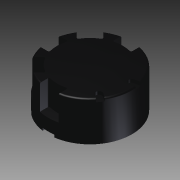
# Autodesk Inventor part: HS13Z-body
Saved by Autodesk Inventor 2011 SP1 (Build 150282100, 282)
## iProperties
Created: 2016-09-01
Part Number: HS13Z-body
Catalog Web Link: www.cadenas.de
Description: HS Series - 6 AMP Single Pole Standard Size Rotaries -body-
Vendor: NKKSWITCHES
Document SubType Name: Modeling
Designer: psAdmin
Manufacturer: NKKSWITCHES
Mass: 13.0423 g
Surface Area: 39.466 cm^2
Volume: 13.0423 cm^3
Density: 1 g/cm^3
Category: PARTsolutions
Company: NKKSWITCHES
Title: HS13Z-body
Author: Cadenas PARTsolutions
PSOL_IDENT_0: {$CADENAS_DATA\23d-libs\nkkswitches\rotary\hs_12_amp\parts\hs_6amp_body.prj},214 {VTYP=3D},{NB=HS13Z
PSOL_IDENT_1: -body},{LINA=HS13Z-body},{NN=HS Series - 6 AMP Single Pole Standard Size Rotaries -body},{DATE=22.09
PSOL_IDENT_2: .2015 06:04:15},{GEOMDATE=26.03.2009 11:48:00},{VERSION=},{LINEID=30},{LINESUBID=-1},{WBVAR=}  {NB=H
PSOL_IDENT_3: S13Z-body},{LINA=HS13Z-body},{KT=DUMMY},{PN=HS13Z},{SRS=HS},{MDL=HS13Z}
NN: HS Series - 6 AMP Single Pole Standard Size Rotaries -body
NB: HS13Z-body
NBSYN: $PN.-body
LINA: HS13Z-body
PN: HS13Z
SRS: HS
MDL: HS13Z
SUPPLIER: NKKSWITCHES
ARTICLENO: HS13Z-body
BOMINFO: HS13Z-body
CREATOR: CADENAS GmbH
Autodesk Inventor part; units mm, degrees
sketch "Sketch_1" plane through (0, 0, 0) normal (1, 0, 0) x (0, 1, 0)
  line L0 (-16.002, 0) -> (0, 0)
  line L1 (0, 0) -> (0, -16.3703)
  arc A0 (-0.635, -17.0053) -> (0, -16.3703) centre (-0.635, -16.3703) ccw
  line L2 (-0.635, -17.0053) -> (-16.002, -17.0053)
  line L3 (-16.002, -17.0053) -> (-16.002, 0)
  line L4 (-16.002, 0) -> (0, 0)
  constraints: 10 end point, 2 point on circle, 1 centre point
revolve "Revolution1" add sketch "Sketch_1" angle 360 about axis through (0, -16.002, 0) along (0, -1, 0)
sketch "Sketch_2" plane through (0, 0, 0) normal (0, 1, 0) x (-1, 0, 0)
  circle A0 centre (0, 0) radius 21.59
  line L0 (17.78, -3.81) -> (13.4434, -3.81)
  arc A1 (12.9501, -3.1808) -> (13.4434, -3.81) centre (13.4434, -3.302) ccw
  arc A2 (12.9501, -3.1808) -> (12.9501, 3.1808) centre (0, 0) ccw
  arc A3 (13.4434, 3.81) -> (12.9501, 3.1808) centre (13.4434, 3.302) ccw
  line L1 (13.4434, 3.81) -> (17.78, 3.81)
  arc A4 (17.78, 3.81) -> (15.2664, 9.8783) centre (0, 0) ccw
  line L2 (15.2664, 9.8783) -> (12.2, 6.8119)
  arc A5 (11.4063, 6.9079) -> (12.2, 6.8119) centre (11.8408, 7.1711) ccw
  arc A6 (11.4063, 6.9079) -> (6.9079, 11.4063) centre (0, 0) ccw
  arc A7 (6.8119, 12.2) -> (6.9079, 11.4063) centre (7.1711, 11.8408) ccw
  line L3 (6.8119, 12.2) -> (9.8783, 15.2664)
  arc A8 (9.8783, 15.2664) -> (3.81, 17.78) centre (0, 0) ccw
  line L4 (3.81, 17.78) -> (3.81, 13.4434)
  arc A9 (3.1808, 12.9501) -> (3.81, 13.4434) centre (3.302, 13.4434) ccw
  arc A10 (3.1808, 12.9501) -> (-3.1808, 12.9501) centre (0, 0) ccw
  arc A11 (-3.81, 13.4434) -> (-3.1808, 12.9501) centre (-3.302, 13.4434) ccw
  line L5 (-3.81, 13.4434) -> (-3.81, 17.78)
  arc A12 (-3.81, 17.78) -> (-3.81, -17.78) centre (0, 0) ccw
  line L6 (-3.81, -17.78) -> (-3.81, -13.4434)
  arc A13 (-3.1808, -12.9501) -> (-3.81, -13.4434) centre (-3.302, -13.4434) ccw
  arc A14 (-3.1808, -12.9501) -> (3.1808, -12.9501) centre (0, 0) ccw
  arc A15 (3.81, -13.4434) -> (3.1808, -12.9501) centre (3.302, -13.4434) ccw
  line L7 (3.81, -13.4434) -> (3.81, -17.78)
  arc A16 (3.81, -17.78) -> (9.8783, -15.2664) centre (0, 0) ccw
  line L8 (9.8783, -15.2664) -> (6.8119, -12.2)
  arc A17 (6.9079, -11.4063) -> (6.8119, -12.2) centre (7.1711, -11.8408) ccw
  arc A18 (6.9079, -11.4063) -> (11.4063, -6.9079) centre (0, 0) ccw
  arc A19 (12.2, -6.8119) -> (11.4063, -6.9079) centre (11.8408, -7.1711) ccw
  line L9 (12.2, -6.8119) -> (15.2664, -9.8783)
  arc A20 (15.2664, -9.8783) -> (17.78, -3.81) centre (0, 0) ccw
  constraints: 40 point on circle, 21 centre point, 20 end point
extrude "Extrusion1" cut sketch "Sketch_2" against normal blind 10.16
sketch "Sketch_3" plane through (0, 0, 0) normal (0, 1, 0) x (-1, 0, 0)
  circle A0 centre (0, 0) radius 20.4599
  arc A1 (-17.2893, -4.3382) -> (-13.8361, 11.2385) centre (0, 0) ccw
  line L0 (-13.8361, 11.2385) -> (-11.2363, 9.4181)
  arc A2 (-12.6468, 7.305) -> (-11.2363, 9.4181) centre (-11.9823, 8.3888) ccw
  line L1 (-12.6468, 7.305) -> (-15.293, 9.1579)
  arc A3 (-15.293, 9.1579) -> (-17.7304, -1.8368) centre (0, 0) ccw
  line L2 (-17.7304, -1.8368) -> (-14.6049, -1.2856)
  arc A4 (-14.1081, -3.7772) -> (-14.6049, -1.2856) centre (-14.4046, -2.541) ccw
  line L3 (-14.1081, -3.7772) -> (-17.2893, -4.3382)
  constraints: 8 end point, 8 point on circle, 5 centre point
extrude "Extrusion2" cut sketch "Sketch_3" against normal blind 1.27
sketch "Sketch_4" plane through (0, -16.002, 0) normal (0, 1, 0) x (1, 0, 0)
  circle A0 centre (0, 0) radius 21.59
  line L0 (-17.78, 2.4003) -> (-13.1172, 2.4003)
  arc A1 (-13.1172, 2.4003) -> (-13.1172, -2.4003) centre (0, 0) ccw
  line L1 (-13.1172, -2.4003) -> (-17.78, -2.4003)
  arc A2 (-17.78, -2.4003) -> (-14.2696, -10.8751) centre (0, 0) ccw
  line L2 (-14.2696, -10.8751) -> (-10.9725, -7.578)
  arc A3 (-10.9725, -7.578) -> (-7.578, -10.9725) centre (0, 0) ccw
  line L3 (-7.578, -10.9725) -> (-10.8751, -14.2696)
  arc A4 (-10.8751, -14.2696) -> (-2.4003, -17.78) centre (0, 0) ccw
  line L4 (-2.4003, -17.78) -> (-2.4003, -13.1172)
  arc A5 (-2.4003, -13.1172) -> (2.4003, -13.1172) centre (0, 0) ccw
  line L5 (2.4003, -13.1172) -> (2.4003, -17.78)
  arc A6 (2.4003, -17.78) -> (2.4003, 17.78) centre (0, 0) ccw
  line L6 (2.4003, 17.78) -> (2.4003, 13.1172)
  arc A7 (2.4003, 13.1172) -> (-2.4003, 13.1172) centre (0, 0) ccw
  line L7 (-2.4003, 13.1172) -> (-2.4003, 17.78)
  arc A8 (-2.4003, 17.78) -> (-10.8751, 14.2696) centre (0, 0) ccw
  line L8 (-10.8751, 14.2696) -> (-7.578, 10.9725)
  arc A9 (-7.578, 10.9725) -> (-10.9725, 7.578) centre (0, 0) ccw
  line L9 (-10.9725, 7.578) -> (-14.2696, 10.8751)
  arc A10 (-14.2696, 10.8751) -> (-17.78, 2.4003) centre (0, 0) ccw
  constraints: 20 end point, 20 point on circle, 11 centre point
extrude "Extrusion3" cut sketch "Sketch_4" along normal blind 1.016
sketch "Sketch_8" plane through (0, 0, 0) normal (0, 1, 0) x (-1, 0, 0)
  arc A0 (3.6802, 0.9861) -> (0.9861, 3.6802) centre (0, 0) ccw
  line L0 (0.9861, 3.6802) -> (-3.6802, -0.9861)
  arc A1 (-3.6802, -0.9861) -> (-0.9861, -3.6802) centre (0, 0) ccw
  line L1 (-0.9861, -3.6802) -> (3.6802, 0.9861)
  constraints: 4 end point, 4 point on circle, 2 centre point
extrude "Extrusion4" add sketch "Sketch_8" against normal blind 17.78
ref_plane "to_dummy_XY" through (0, 0, 0) normal (0, -1, 0) x (1, 0, 0)
ref_plane "to_dummy_YZ" through (0, 0, 0) normal (1, 0, 0) x (0, 0, 1)
ref_plane "to_dummy_ZX" through (0, 0, 0) normal (0, 0, 1) x (0, -1, 0)
ref_plane "to_shaft_XY" through (0, 0, 0) normal (0, -1, 0) x (1, 0, 0)
ref_plane "to_shaft_YZ" through (0, 0, 0) normal (1, 0, 0) x (0, 0, 1)
ref_plane "to_shaft_ZX" through (0, 0, 0) normal (0, 0, 1) x (0, -1, 0)
ref_plane "to_trmnls_XY" through (0, -14.986, 0) normal (0, 1, 0) x (1, 0, 0)
ref_plane "to_trmnls_YZ" through (0, -14.986, 0) normal (1, 0, 0) x (0, 0, -1)
ref_plane "to_trmnls_ZX" through (0, -14.986, 0) normal (0, 0, -1) x (0, 1, 0)
body "Solid1"
